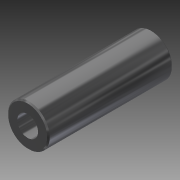
# Autodesk Inventor part: lexan top bolt spacer
Saved by Autodesk Inventor 2011 (Build 150239000, 239)
## iProperties
Category: Chassis
Company: Autodesk Inc.
Created: 2011-01-10
Part Number: lexan top bolt spacer
Document SubType Name: Modeling
Designer: Autodesk Inc.
Density: 1 g/cm^3
Catalog Web Link: http://www.andymark.com/productdetails.asp?productcode=am-0754
Vendor: Andy Mark Inc.
Author: Autodesk Inc.
Autodesk Inventor part; units mm, degrees
ref_plane "YZ Plane" through (0, 0, 0) normal (1, 0, 0) x (0, 1, 0)
ref_plane "XZ Plane" through (0, 0, 0) normal (0, 1, 0) x (-1, 0, 0)
ref_plane "XY Plane" through (0, 0, 0) normal (0, 0, 1) x (1, 0, 0)
sketch "Sketch1" plane through (0, 0, 0) normal (0, 0, 1) x (1, 0, 0)
  circle A0 centre (0, 0) radius 3.175
  circle A1 centre (0, 0) radius 6.35
  dimension "d0" = 6.35
  dimension "d1" = 12.7
  constraints: 2 centre point, 2 coincident
  measures "d0" diameter of A0
  measures "d1" diameter of A1
extrude "Extrusion1" add sketch "Sketch1" against normal blind 38.1
chamfer "Chamfer1" distance 0.3969 angle 45 2 edges at (-6.35, 0, 0) (-6.35, 0, -38.1)
body "Solid1"
